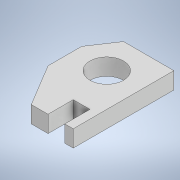
# Autodesk Inventor part: InclinedSupport
Saved by Autodesk Inventor 2022.2 (Build 262287030, 287C)
## iProperties
Created: 2023-02-06
Part Number: InclinedSupport
Material: Generic
Document SubType Name: Modeling
Designer: jak27277
Density: 1 g/cm^3
Appearance: Default
Author: jak27277
Autodesk Inventor part; units mm, degrees
ref_plane "YZ Plane" through (0, 0, 0) normal (1, 0, 0) x (0, 1, 0)
ref_plane "XZ Plane" through (0, 0, 0) normal (0, 1, 0) x (-1, 0, 0)
ref_plane "XY Plane" through (0, 0, 0) normal (0, 0, 1) x (1, 0, 0)
sketch "Sketch1" plane through (0, 0, 0) normal (0, 1, 0) x (-1, 0, 0)
  circle A0 centre (0, 0) radius 12.7
  line L0 (-25.4, -25.4) -> (12.7, -25.4)
  line L1 (12.7, -25.4) -> (25.4, -6.35)
  line L2 (25.4, -6.35) -> (25.4, 19.05)
  line L3 (25.4, 19.05) -> (6.35, 50.8)
  line L4 (6.35, 50.8) -> (-6.35, 50.8)
  line L5 (-6.35, 50.8) -> (-6.35, 31.75)
  line L6 (-6.35, 31.75) -> (-19.05, 31.75)
  line L7 (-19.05, 31.75) -> (-19.05, 50.8)
  line L8 (-19.05, 50.8) -> (-25.4, 50.8)
  line L9 (-25.4, 50.8) -> (-25.4, -25.4)
  dimension "d0" = 25.4
  dimension "d1" = 25.4
  dimension "d2" = 25.4
  dimension "d3" = 19.05
  dimension "d4" = 25.4
  dimension "d5" = 38.1
  dimension "d6" = 50.8
  dimension "d8" = 31.75
  dimension "d9" = 6.35
  dimension "d10" = 19.05
  dimension "d11" = 12.7
  dimension "d12" = 76.2
  constraints: 20 end point, 5 perpendicular, 2 point on line, 1 centre point, 1 coincident, 1 horizontal, 1 parallel
  measures "d0" diameter of A0
  measures "d1" distance from line of L0 point (0, 0)
  measures "d2" distance from line of L9 point (0, 0)
  measures "d3" vertical distance of L0.end L1.end
  measures "d4" distance of L1.end L2.end
  measures "d5" distance of L0.start L0.end
  measures "d6" distance between parallel lines of L9 L2
  measures "d8" distance of L8.end L3.end
  measures "d9" distance of L7.end L8.end
  measures "d10" distance of L6.end L7.end
  measures "d11" distance of L5.end L6.end
  measures "d12" distance of L8.end L0.start
extrude "Extrusion1" add sketch "Sketch1" along normal blind 12.7
body "Solid1"
